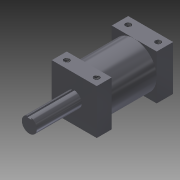
# Autodesk Inventor part: hack_p60
Saved by Autodesk Inventor 2011 (Build 150239000, 239)
## iProperties
Created: 2013-01-17
Part Number: hack_p60
Document SubType Name: Modeling
Designer: Christopher
Density: 1 g/cm^3
Author: Christopher
Autodesk Inventor part; units mm, degrees
ref_plane "YZ Plane" through (0, 0, 0) normal (1, 0, 0) x (0, 1, 0)
ref_plane "XZ Plane" through (0, 0, 0) normal (0, 1, 0) x (-1, 0, 0)
ref_plane "XY Plane" through (0, 0, 0) normal (0, 0, 1) x (1, 0, 0)
sketch "Sketch1" plane through (0, 0, 0) normal (0, 0, 1) x (1, 0, 0)
  line L0 (0, 0) -> (38.1, 0)
  line L1 (38.1, 0) -> (38.1, 38.1)
  line L2 (38.1, 38.1) -> (0, 38.1)
  line L3 (0, 38.1) -> (0, 0)
  circle A0 centre (19.05, 19.05) radius 6.35
  line L4 (20.6375, 23.8125) -> (17.4625, 23.8125)
  line L5 (17.4625, 25.4) -> (20.6375, 25.4)
  line L6 (20.6375, 23.8125) -> (20.6375, 25.4)
  line L7 (17.4625, 23.8125) -> (17.4625, 25.4)
  circle A1 centre (19.05, 19.05) radius 19.05
  point P0 (19.05, 0)
  point P1 (0, 19.05)
  point P2 (19.05, 23.8125)
  dimension "d0" = 38.1
  dimension "d1" = 38.1
  dimension "d2" = 12.7
  dimension "d3" = 3.175
  constraints: 16 end point, 3 midpoint, 3 parallel, 2 centre point, 2 perpendicular, 1 coincident, 1 horizontal, 1 horizontal alignment, 1 tangent, 1 vertical alignment
  measures "d0" distance of L2.end L1.end
  measures "d1" distance of L1.end L0.end
  measures "d2" diameter of A0
  measures "d3" distance of L4.start L4.end
extrude "Extrusion1" add sketch "Sketch1" along normal blind 12.7 contours L3 A1 L0 | A1 L1 L0 | A1 | L3 L2 A1 | A1 L2 L1 | A0 L7 L4 L6 | L6 L4 L7 A0
extrude "Extrusion2" add sketch "Sketch1" along normal blind 50.8 contours A0 L7 L4 L6 | L6 L4 L7 A0
extrude "Extrusion3" cut sketch "Sketch1" along normal blind 50.8 contours L6 L4 L7 A0 | A0 L5 L6 | L7 L5 A0 picked at (19.05, 24.3417)
extrude "Extrusion4" add sketch "Sketch1" against normal blind 38.1 contours A1
sketch "Sketch2" plane through (19.05, 19.05, -38.1) normal (0, 0, -1) x (-1, 0, 0)
  arc A0 (-1.5875, 6.1484) -> (1.5875, 6.1484) centre (0, 0) ccw projected
  line L0 (-1.5875, 6.1484) -> (-1.5875, 6.35) projected
  line L1 (-1.5875, 6.35) -> (1.5875, 6.35) projected
  line L2 (1.5875, 6.35) -> (1.5875, 6.1484) projected
  circle A1 centre (0, 0) radius 19.05 projected
  line L3 (-19.05, 19.05) -> (19.05, 19.05)
  line L4 (19.05, 19.05) -> (19.05, -19.05)
  line L5 (19.05, -19.05) -> (-19.05, -19.05)
  line L6 (-19.05, -19.05) -> (-19.05, 19.05)
  constraints: 8 end point, 2 parallel, 2 tangent, 1 horizontal, 1 perpendicular
extrude "Extrusion5" add sketch "Sketch2" along normal blind 13.97
sketch "Sketch3" plane through (0, 38.1, 12.7) normal (0, 1, 0) x (1, 0, 0)
  line L0 (0, 0) -> (38.1, 0) projected
  line L1 (0, 12.7) -> (0, 0) projected
  point P0 (31.75, 6.35)
  point P1 (6.35, 6.35)
  point P2 (6.35, 58.42)
  point P3 (31.75, 58.42)
  point P4 (0, 64.77)
  dimension "d15" = 6.35
  dimension "d16" = 25.4
  dimension "d17" = 6.35
  dimension "d18" = 6.35
  constraints: 2 horizontal alignment, 2 vertical alignment
  measures "d15" distance from line of L0 point (31.75, 6.35)
  measures "d16" distance of point (6.35, 6.35) point (31.75, 6.35)
  measures "d17" distance from line of L1 point (6.35, 6.35)
  measures "d18" horizontal distance of point (0, 64.77) point (6.35, 58.42)
hole "Hole1" at (31.75, 38.1, 6.35) at (6.35, 38.1, 6.35) at (6.35, 38.1, -45.72) at (31.75, 38.1, -45.72) direction (0, -1, 0) diameter 4.7625 depth 12.7 tip angle 118
thread "Thread1" size "10-32 UNF" class "2B" standard "ANSI Unified Screw Threads" full length
thread "Thread2" size "10-32 UNF" class "2B" standard "ANSI Unified Screw Threads" full length
thread "Thread3" size "10-24 UNC" class "2B" standard "ANSI Unified Screw Threads" full length
thread "Thread4" size "10-24 UNC" class "2B" standard "ANSI Unified Screw Threads" full length
body "Solid1"
